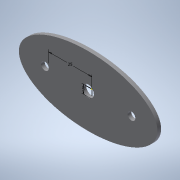
# Autodesk Inventor part: SP58V1 Seguro Pedales
Saved by Autodesk Inventor 2021.2 (Build 252289000, 289)
## iProperties
Created: 2026-10-05
Part Number: SP58V1 Seguro Pedales
Material: Generic
Document SubType Name: Sheet Metal
Designer: nelso
Density: 1 g/cm^3
Sheet Metal Rule: Default_mm
Appearance: Default
Author: nelso
Autodesk Inventor part; units mm, degrees
ref_plane "YZ Plane" through (0, 0, 0) normal (1, 0, 0) x (0, 1, 0)
ref_plane "XZ Plane" through (0, 0, 0) normal (0, 1, 0) x (-1, 0, 0)
ref_plane "XY Plane" through (0, 0, 0) normal (0, 0, 1) x (1, 0, 0)
sketch "Sketch1" plane through (0, 0, 0) normal (0, 1, 0) x (-1, 0, 0)
  ellipse E0 centre (0, 0) end of major axis (-40, 0) minor radius 20
  dimension "d0" = 40
  dimension "d1" = 20
extrude "Plate1" add sketch "Sketch1" along normal blind 2.1
sketch "Sketch2" plane through (0, 2.1, 0) normal (0, 1, 0) x (1, 0, 0)
  line L0 (0, 0) -> (-25, 0)
  line L1 (0, 0) -> (0, 5)
  point P0 (25, 0)
  point P1 (25, 0)
  dimension "d3" = 25
  dimension "d4" = 5
  constraints: 4 end point, 3 coincident, 2 symmetric about line, 1 horizontal, 1 vertical
  measures "d3" distance of L0.start L0.end
  measures "d4" distance of L0.start L1.end
hole "Hole1" at (0, 2.1, 0) direction (0, -1, 0) diameter 6.6 depth 2.1 clearance for "Countersunk Flat Head Screw ISO 2009/7046" size "M6" standard "ISO"
hole "Hole2" at (-25, 2.1, 0) at (25, 2.1, 0) direction (0, -1, 0) diameter 4.5 depth 2.1 clearance for "Countersunk Flat Head Screw ISO 2009/7046" size "M4" standard "ISO"
equation "\"d10\" = Thickness"
equation "\"d17\" = Thickness"
equation "\"d2\" = Thickness"
equation "\"BendReliefWidth\" = Thickness"
equation "\"BendReliefDepth\" = 0.5 * Thickness"
equation "\"CornerReliefSize\" = 4 * Thickness"
equation "\"MinimumRemnant\" = 2 * Thickness"
equation "\"TransitionRadius\" = BendRadius"
equation "\"JacobiRadiusSize\" = BendRadius"
equation "\"GapSize\" = Thickness"
equation "\"Thickness\" = 2.1"
equation "\"BendRadius\" = 1.512"
body "Solid1"
